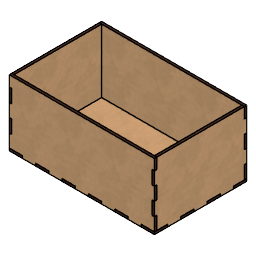
finger joint box (Autodesk Fusion 360 design; units mm, degrees)
part number: 2026-07-23-17-33-07-436
Autodesk Fusion 360 part; units mm, degrees
sketch "BottomPanelSketch" plane through (0, 0, 0) normal (0, 1, 0) x (1, 0, 0)
  line L0 (0, 0) -> (1100, 0)
  line L1 (1100, 0) -> (1100, 700)
  line L2 (1100, 700) -> (0, 700)
  line L3 (0, 700) -> (0, 0)
  dimension "d12" = 1100
  dimension "d13" = 700
  constraint horizontal L0
  constraint vertical L1
  constraint horizontal L2
  constraint vertical L3
  constraint coincident L0.start L3.end
  measures "d12" distance of L0.start L0.end
  measures "d13" distance of L0.start L2.end
extrude "Extrude1" add sketch "BottomPanelSketch" along normal blind 18 makes body 1
sketch "BottomPanelFrontFingersSketch" plane through (0, 0, 0) normal (0, 0, 1) x (1, 0, 0)
  line L0 (0, 0) -> (1100, 0)
  line L1 (1100, 0) -> (1100, 18)
  line L2 (1100, 18) -> (0, 18)
  line L3 (0, 18) -> (0, 0)
  line L4 (100, 0) -> (200, 0)
  line L5 (200, 0) -> (200, 18)
  line L6 (200, 18) -> (100, 18)
  line L7 (100, 18) -> (100, 0)
  dimension "d16" = 100
  dimension "d17" = 100
  constraint horizontal L4
  constraint vertical L5
  constraint horizontal L6
  constraint vertical L7
  constraint coincident L2 L5.end
  constraint coincident L0 L4.start
  measures "d16" distance of L5.end L6.end
  measures "d17" distance of L3 L7
extrude "Extrude2" cut sketch "BottomPanelFrontFingersSketch" against normal blind 18 contours L0 L2 L4 L5 L6 L7 bodies 1
pattern_linear "R-Pattern1" count 5 spacing 200 along (1, 0, 0) of "Extrude2"
sketch "FrontPanelSketch" plane through (0, 0, 0) normal (0, 0, 1) x (1, 0, 0)
  line L0 (0, 0) -> (1100, 0)
  line L1 (1100, 0) -> (1100, 500)
  line L2 (1100, 500) -> (0, 500)
  line L3 (0, 500) -> (0, 0)
  dimension "d24" = 1100
  dimension "d25" = 500
  constraint horizontal L0
  constraint vertical L1
  constraint horizontal L2
  constraint vertical L3
  constraint coincident L0.start L3.end
  measures "d24" distance of L0.start L0.end
  measures "d25" distance of L0.start L2.end
extrude "Extrude3" add sketch "FrontPanelSketch" against normal blind 18 separate body makes body 2
combine "Combine1" operation cut target body 2 tool bodies 1 keep tools
sketch "BackPanelSketch" plane through (0, 0, 0) normal (-1, 0, 0) x (0, 0, 1)
  line L0 (-18, 18) -> (0, 18)
  line L1 (0, 18) -> (0, 500)
  line L2 (0, 500) -> (-18, 500)
  line L3 (-18, 500) -> (-18, 18)
  line L4 (0, 118) -> (-18, 118)
  line L5 (-18, 118) -> (-18, 218)
  line L6 (-18, 218) -> (0, 218)
  line L7 (0, 218) -> (0, 118)
  dimension "d28" = 100
  dimension "d29" = 100
  constraint horizontal L4
  constraint vertical L5
  constraint horizontal L6
  constraint vertical L7
  constraint coincident L3 L5.end
  constraint coincident L1 L4.start
  measures "d28" distance of L4.end L5.end
  measures "d29" distance of L0 L4
extrude "Extrude4" cut sketch "BackPanelSketch" against normal blind 18 contours L1 L3 L4 L5 L6 L7 bodies 2
pattern_linear "R-Pattern2" count 2 spacing 200 along (0, 1, 0) of "Extrude4"
extrude "Extrude5" add 1 faces at (572.6667, 312, -18) along direction (0, 0, 1) blind 18 from surface at -682 separate body on bodies 2 makes body 3
combine "Combine2" operation cut target body 1 tool bodies 3 keep tools
sketch "SidePanelFingersSketch" plane through (0, 0, 0) normal (-1, 0, 0) x (0, 0, 1)
  line L0 (-700, 0) -> (0, 0)
  line L1 (0, 0) -> (0, 18)
  line L2 (0, 18) -> (-700, 18)
  line L3 (-700, 18) -> (-700, 0)
  line L4 (-100, 0) -> (-200, 0)
  line L5 (-200, 0) -> (-200, 18)
  line L6 (-200, 18) -> (-100, 18)
  line L7 (-100, 18) -> (-100, 0)
  dimension "d41" = 100
  dimension "d42" = 100
  constraint horizontal L4
  constraint vertical L5
  constraint horizontal L6
  constraint vertical L7
  constraint coincident L2 L5.end
  constraint coincident L0 L4.start
  measures "d41" distance of L5.end L6.end
  measures "d42" distance of L1 L7
extrude "Extrude7" cut sketch "SidePanelFingersSketch" against normal blind 18 contours L0 L2 L4 L5 L6 L7 bodies 1
pattern_linear "R-Pattern3" count 3 spacing 200 along (0, 0, -1) of "Extrude7"
sketch "LeftPanelSketch" plane through (0, 0, 0) normal (-1, 0, 0) x (0, 0, 1)
  line L0 (-700, 500) -> (-700, 418)
  line L1 (-700, 418) -> (-682, 418)
  line L2 (-682, 418) -> (-682, 500)
  line L3 (-682, 500) -> (-700, 500)
  line L4 (0, 0) -> (-700, 0)
  line L5 (-700, 0) -> (-700, 500)
  line L6 (-700, 500) -> (0, 500)
  line L7 (0, 500) -> (0, 0)
  constraint horizontal L4
  constraint vertical L5
  constraint horizontal L6
  constraint vertical L7
  constraint coincident L0.start L3.end
  constraint coincident L4.start L7.end
extrude "Extrude8" add sketch "LeftPanelSketch" against normal blind 18 separate body contours L1 L2 L4 L5 L6 L7 makes body 4
combine "Combine3" operation cut target body 4 tool bodies 3 1 2 keep tools
extrude "Extrude9" add 1 faces at (18, 218, -366.6667) along direction (-1, 0, 0) blind 18 from surface at -1082 separate body on bodies 4 makes body 5
combine "Combine4" operation cut target body 2 tool bodies 5 keep tools
combine "Combine5" operation cut target body 1 tool bodies 5 keep tools
combine "Combine6" operation cut target body 3 tool bodies 5 keep tools
equation "length = 1100 mm"
equation "width = 700 mm"
equation "height = 500 mm"
equation "thickness = 18 mm"
equation "lengthFingers = 5"
equation "widthFingers = 3"
equation "heightFingers = 2"
equation "lengthFingersWidth = length / ( ( lengthFingers * 2 ) + 1 )"
equation "widthFingersWidth = width / ( ( widthFingers * 2 ) + 1 )"
equation "heightFingersWidth = height / ( ( heightFingers * 2 ) + 1 )"
equation "d12 = length"
equation "d13 = width"
equation "d14 = thickness"
equation "d16 = lengthFingersWidth"
equation "d17 = lengthFingersWidth"
equation "d18 = -thickness"
equation "d20 = lengthFingers"
equation "d22 = length - ( lengthFingersWidth * 3 )"
equation "d24 = length"
equation "d25 = height"
equation "d26 = -thickness"
equation "d28 = heightFingersWidth"
equation "d29 = heightFingersWidth"
equation "d30 = -thickness"
equation "d32 = heightFingers"
equation "d34 = height - ( heightFingersWidth * 3 )"
equation "d37 = -thickness"
equation "d41 = widthFingersWidth"
equation "d42 = widthFingersWidth"
equation "d43 = -thickness"
equation "d45 = widthFingers"
equation "d47 = -( width - widthFingersWidth * 3 )"
equation "d49 = -thickness"
equation "d52 = -thickness"
named bodies: "BottomPanel", "FrontPanel", "BackPanel", "LeftPanel", "RightPanel"
